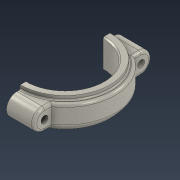
# Autodesk Inventor part: Pokrywa stopy korbowodu
Saved by Autodesk Inventor 2022 (Build 260153000, 153)
## iProperties
Created: 2023-05-22
Part Number: Pokrywa stopy korbowodu
Material: Generic
Document SubType Name: Modeling
Designer: wikto
Density: 1 g/cm^3
Appearance: Steel - Cast
Author: wikto
Autodesk Inventor part; units mm, degrees
ref_plane "YZ Plane" through (0, 0, 0) normal (1, 0, 0) x (0, 1, 0)
ref_plane "XZ Plane" through (0, 0, 0) normal (0, 1, 0) x (-1, 0, 0)
ref_plane "XY Plane" through (0, 0, 0) normal (0, 0, 1) x (1, 0, 0)
sketch "Sketch1" plane through (0, 0, 0) normal (0, 1, 0) x (-1, 0, 0)
  arc A0 (0, 27.5) -> (0, -27.5) centre (0, 0) ccw
  arc A1 (0, 32.5) -> (0, -32.5) centre (0, 0) ccw
  line L0 (0, -32.5) -> (0, -42.5)
  line L1 (0, -42.5) -> (-20, -42.5)
  line L2 (-20, -42.5) -> (-20, -25.6174)
  line L3 (-20, 25.6174) -> (-20, 42.5)
  line L4 (-20, 42.5) -> (0, 42.5)
  line L5 (0, 42.5) -> (0, 32.5)
  line L6 (0, -32.5) -> (0, -27.5)
  line L7 (0, 27.5) -> (0, 32.5)
  arc A2 (-20, 29.9333) -> (-20, -29.9333) centre (0, 0) ccw
  dimension "d0" = 27.5
  dimension "d1" = 32.5
  dimension "d2" = 10
  dimension "d3" = 20
  dimension "d4" = 36
  constraints: 16 end point, 8 point on circle, 4 perpendicular, 4 vertical, 3 centre point, 3 coincident, 3 equal length, 2 point on line, 2 vertical alignment
  measures "d0" radius of A0
  measures "d1" radius of A1
  measures "d2" distance of L0.start L0.end
  measures "d3" distance of L0.end L1.end
  measures "d4" radius of A2
extrude "Extrusion1" add sketch "Sketch1" along normal mid plane 21 contours A0 L6 A1 L7
extrude "Extrusion2" add sketch "Sketch1" along normal mid plane 15 contours A1 L3 L4 L5 | L0 L1 L2 A1 | A1 L2 A2 L3
sketch "Sketch2" plane through (0, -10.5, -27.5) normal (-1, 0, 0) x (0, 0, 1)
  line L0 (0, 21) -> (0, 0) projected
  line L1 (55, 0) -> (55, 21) projected
  point P0 (27.5, 10.5)
  point P1 (-7.5, 10.5)
  point P2 (62.5, 10.5)
  dimension "d9" = 7.5
  dimension "d10" = 7.5
  constraints: 2 horizontal alignment
  measures "d9" distance from line of L0 point (-7.5, 10.5)
  measures "d10" distance from line of L1 point (62.5, 10.5)
hole "Hole1" at (0, 0, -35) at (0, 0, 35) direction (1, 0, 0) diameter 5 end through all
full round fillet "Full Round Fillet1" first side at (9.2593, 7.5, 38.8519) centre faces at (13.3333, -2.5, -42.5) second side at (9.2593, -7.5, 38.8519)
full round fillet "Full Round Fillet2" first side at (9.2593, -7.5, 38.8519) centre faces at (6.6667, -2.5, 42.5) second side at (9.2593, 7.5, 38.8519)
fillet "Fillet1" radius 2 10 edges at (36, -7.5, 0) (20, 5.3033, 40.3033) (20, -5.3033, 40.3033) (20, 7.5, 32.4667) (20, -7.5, 32.4667) (36, 7.5, 0) (20, -7.5, -32.4667) (20, 7.5, -32.4667) (20, 5.3033, -40.3033) (20, -5.3033, -40.3033)
chamfer "Chamfer1" distance 1 angle 45 2 edges at (27.5, -10.5, 0) (27.5, 10.5, 0)
fillet "Fillet2" radius 1 2 edges at (32.5, 7.5, 0) (32.5, -7.5, 0)
body "Solid1"
